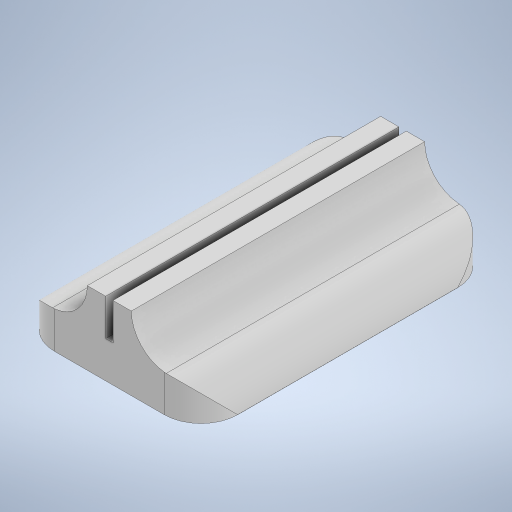
# Autodesk Inventor part: CalibrationWallMounts
Saved by Autodesk Inventor 2024.2 (Build 282272000, 272)
## iProperties
Created: 2024-05-02
Part Number: CalibrationWallMounts
Material: Generic
Document SubType Name: Modeling
Designer: ringl
Density: 1 g/cm^3
Appearance: Default
Author: ringl
Autodesk Inventor part; units mm, degrees
ref_plane "YZ Plane" through (0, 0, 0) normal (1, 0, 0) x (0, 1, 0)
ref_plane "XZ Plane" through (0, 0, 0) normal (0, 1, 0) x (-1, 0, 0)
ref_plane "XY Plane" through (0, 0, 0) normal (0, 0, 1) x (1, 0, 0)
sketch "Sketch1" plane through (0, 0, 0) normal (0, 1, 0) x (-1, 0, 0)
  line L0 (0, 0) -> (50, 0)
  line L1 (50, 0) -> (50, -80)
  line L2 (50, -80) -> (0, -80)
  line L3 (0, -80) -> (0, 0)
  dimension "d0" = 50
  dimension "d1" = 80
  constraints: 8 end point, 2 parallel, 1 horizontal, 1 perpendicular
  measures "d0" distance of L1.end L2.end
  measures "d1" distance of L0.end L1.end
extrude "Extrusion1" add sketch "Sketch1" along normal blind 10
sketch "Sketch2" plane through (0, 10, 0) normal (0, 1, 0) x (1, 0, 0)
  line L0 (-31, 0) -> (-26, 0)
  line L1 (-26, 0) -> (-26, 80)
  line L2 (-26, 80) -> (-31, 80)
  line L3 (-31, 80) -> (-31, 0)
  line L4 (-50, 0) -> (0, 0) projected
  line L5 (0, 80) -> (-50, 80) projected
  line L6 (-19, 0) -> (-24, 0)
  line L7 (-24, 0) -> (-24, 80)
  line L8 (-24, 80) -> (-19, 80)
  line L9 (-19, 80) -> (-19, 0)
  line L10 (0, 0) -> (0, 80) projected
  dimension "d7" = 5
  dimension "d8" = 5
  dimension "d9" = 2
  dimension "d10" = 19
  constraints: 16 end point, 4 parallel, 2 horizontal, 2 perpendicular, 2 point on line
  measures "d7" distance between parallel lines of L7 L9
  measures "d8" distance between parallel lines of L3 L1
  measures "d9" distance between parallel lines of L7 L1
  measures "d10" distance between parallel lines of L10 L9
extrude "Extrusion2" add sketch "Sketch2" along normal blind 10 contours L3 L2 L1 L0 | L7 L5 L9 L4
fillet "Fillet1" radius 10 2 edges at (-19, 10, -40) (-31, 10, -40)
fillet "Fillet2" radius 10 6 edges at (0, 10, -40) (0, 5, -80) (-50, 5, -80) (-50, 5, 0) (0, 5, 0) (-50, 10, -40)
body "Solid1"
